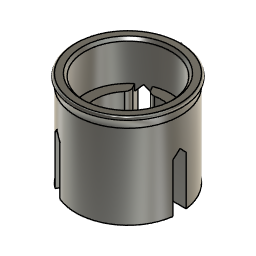
FOI adapter v2 (Autodesk Fusion 360 design; units mm, degrees)
Autodesk Fusion 360 part; units mm, degrees
sketch "Sketch1" plane through (0, 0, 0) normal (0, 0, 1) x (1, 0, 0)
  circle A0 centre (0, 0) radius 7.95
  dimension "d1" = 15.9
  constraint coincident A0.centre origin
  measures "d1" diameter of A0
extrude "Extrude1" add sketch "Sketch1" along normal blind 13.5
sketch "Sketch2" plane through (0, 0, 13.5) normal (0, 0, 1) x (-1, 0, 0)
  circle A0 centre (0, 0) radius 7.95
  circle A1 centre (0, 0) radius 5.075
  dimension "d4" = 10.15
  constraint coincident A0.centre A1.centre
  measures "d4" diameter of A1
extrude "Extrude2" cut sketch "Sketch2" against normal blind 20.505 contours A1
sketch "Sketch3" plane through (0, 0, 13.5) normal (0, 0, 1) x (-1, 0, 0)
  circle A0 centre (0, 0) radius 5.075
  circle A1 centre (0, 0) radius 7.95
  circle A2 centre (0, 0) radius 6.575
  dimension "d7" = 13.15
  constraint coincident A0.centre A1.centre
  measures "d7" diameter of A2
extrude "Extrude3" cut sketch "Sketch3" against normal blind 6 contours A2
extrude "Extrude4" add 1 faces at (6.9432, -0.6471, 0) along direction (0, 0, -1) blind 1
sketch "Sketch4" plane through (0, 0, 0) normal (1, 0, 0) x (0, 1, 0)
  line L0 (-7.95, -1) -> (7.95, -1)
  line L1 (7.95, 13.5) -> (-7.95, 13.5)
  line L2 (7.95, 13.5) -> (8.45, 13.5)
  line L3 (8.45, 13.5) -> (7.45, 11.7679)
  line L4 (8.45, 13.5) -> (10.95, 13.5) construction
  line L5 (7.95, 13.5) -> (7.95, 12.634)
  dimension "d12" = 0.5
  dimension "d13" = 120
  dimension "d14" = 2
  constraint coincident L1.start L2.start
  constraint parallel L1 L2
  constraint horizontal L4
  constraint coincident L3 L5.end
  constraint perpendicular L2 L5
  measures "d12" distance of L1.start L2.end
  measures "d13" angle of L3 L4
  measures "d14" distance of L2.end L3.end
revolve "Revolve1" add sketch "Sketch4" angle 360 about axis through (0, 0, 0) along (0, 0, 1)
fillet "Fillet1" radius 3 1 edges at (-7.412, 2.8748, 12.634)
fillet "Fillet2" radius 0.3 1 edges at (-7.8782, 3.0557, 13.5)
sketch "Sketch5" plane through (0, 0, -1) normal (0, 0, -1) x (1, 0, 0)
  circle A0 centre (0, 0) radius 5.075
  circle A1 centre (0, 0) radius 7.95
  line L0 (12.0081, -1) -> (12.0081, 1.0091)
  line L1 (12.0081, 1.0091) -> (4.9737, 1.0091)
  line L2 (0, 0) -> (12.0081, -1) construction
  line L3 (12.0081, 1.0091) -> (0, 0) construction
  line L4 (4.9755, -1) -> (12.0081, -1)
  line L5 (-6.8779, 9.8948) -> (-3.3607, 3.8028)
  line L6 (-1.6217, 4.8089) -> (-5.138, 10.8993)
  line L7 (-5.138, 10.8993) -> (-6.8779, 9.8948)
  line L8 (-5.1302, -10.9039) -> (-1.613, -4.8119)
  line L9 (-3.3538, -3.8089) -> (-6.8701, -9.8993)
  line L10 (-6.8701, -9.8993) -> (-5.1302, -10.9039)
  dimension "d22" = 360
  constraint horizontal L1
  constraint coincident A0.centre L3
  constraint coincident A0.centre A1.centre
  constraint coincident A0 L1.end
  constraint coincident L2 A0.centre
  constraint coincident A0 L4.start
extrude "Extrude5" cut sketch "Sketch5" against normal blind 8.5 contours A0 A1 L1 L4 | A0 A1 L5 L6 | A0 A1 L8 L9
chamfer "Chamfer1" distance 1 angle 45 6 edges at (7.1927, 1, 7.5) (7.1914, -1.0091, 7.5) (-4.4696, -5.7234, 7.5) (-4.4624, 5.729, 7.5) (-2.7218, 6.7325, 7.5) (-2.7303, -6.729, 7.5)
fillet "Fillet3" radius 1 6 edges at (4.9755, 1, 3.25) (4.9737, -1.0091, 3.25) (-1.6217, -4.8089, 3.25) (-1.613, 4.8119, 3.25) (-3.3538, 3.8089, 3.25) (-3.3607, -3.8028, 3.25)
chamfer "Chamfer2" distance 0.4 angle 45 1 edges at (6.1301, -2.3776, 13.5)
equation "d13 = 90.0 deg + 30 deg"
